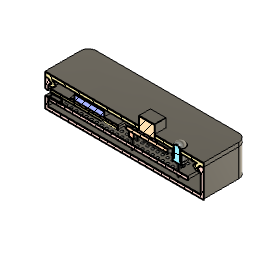
co2-sensor-d1-mini (Autodesk Fusion 360 design; units mm, degrees)
Autodesk Fusion 360 part; units mm, degrees
(part 1 of 2)
sketch "board" plane through (0, 0, 0) normal (0, 0, 1) x (1, 0, 0) in component "Board"
  line L0 (35, 15) -> (-35, 15)
  line L1 (-35, 15) -> (-35, -15)
  line L2 (-35, -15) -> (35, -15)
  line L3 (35, -15) -> (35, 15)
  line L4 (35, 15) -> (-35, -15) construction
  line L5 (-35, 15) -> (35, -15) construction
  dimension "d4" = 70
  dimension "d5" = 30
  constraint horizontal L0
  constraint perpendicular L0 L1
  constraint parallel L0 L2
  constraint parallel L1 L3
  constraint coincident L4 origin
  constraint coincident L5 origin
  measures "d4" distance of L1.end L2.end
  measures "d5" distance of L0.end L1.end
extrude "Extrude1" add sketch "board" along normal blind 1.5 makes body 1 in component "Board"
sketch "holes" plane through (0, 0, 1.5) normal (0, 0, 1) x (-1, 0, 0) in component "Board"
  line L0 (-35, 15) -> (-35, -15)
  line L1 (-35, -15) -> (35, -15)
  line L2 (35, -15) -> (35, 15)
  line L3 (35, 15) -> (-35, 15)
  line L4 (-29.5, -11.5) -> (29.5, -11.5) construction
  line L5 (29.5, -11.5) -> (29.5, 11.5) construction
  line L6 (29.5, 11.5) -> (-29.5, 11.5) construction
  line L7 (-29.5, 11.5) -> (-29.5, -11.5) construction
  line L8 (-29.5, -11.5) -> (29.5, 11.5) construction
  line L9 (29.5, -11.5) -> (-29.5, 11.5) construction
  line L10 (-33, -13.1) -> (33, -13.1) construction
  line L11 (33, -13.1) -> (33, 13.1) construction
  line L12 (33, 13.1) -> (-33, 13.1) construction
  line L13 (-33, 13.1) -> (-33, -13.1) construction
  line L14 (-33, -13.1) -> (33, 13.1) construction
  line L15 (33, -13.1) -> (-33, 13.1) construction
  circle A0 centre (33, -13.1) radius 1.2
  circle A1 centre (29.5, -11.5) radius 0.7
  dimension "d13" = 59
  dimension "d14" = 23
  dimension "d15" = 66
  dimension "d16" = 26.2
  dimension "d17" = 2.4
  dimension "d18" = 1.4
  constraint horizontal L4
  constraint perpendicular L4 L5
  constraint parallel L4 L6
  constraint parallel L5 L7
  constraint coincident L8 origin
  constraint coincident L9 origin
  constraint horizontal L10
  constraint perpendicular L10 L11
  constraint parallel L10 L12
  constraint parallel L11 L13
  constraint coincident L14 origin
  constraint coincident L15 origin
  constraint coincident L10.end L11.start
  constraint coincident L4.end L5.start
  measures "d13" distance of L5.end L6.end
  measures "d14" distance of L4.end L5.end
  measures "d15" distance of L11.end L12.end
  measures "d16" distance of L10.end L11.end
  measures "d17" diameter of A0
  measures "d18" diameter of A1
extrude "Extrude2" cut sketch "holes" against normal through all contours A0 bodies 1 in component "Board"
pattern_linear "R-Pattern1" count 2 spacing 66 along (1, 0, 0) count 2 spacing 26.2 along (0, -1, 0) of "Extrude2" in component "Board"
extrude "Extrude3" cut sketch "holes" against normal through all contours A1 bodies 1 in component "Board"
pattern_linear "R-Pattern2" count 24 spacing 2.5652 along (1, 0, 0) count 10 spacing 2.5556 along (0, -1, 0) of "Extrude3" in component "Board"
sketch "base" plane through (0, 0, 0) normal (0, 0, 1) x (1, 0, 0) in component "D1 Mini"
  line L0 (17.075, 12.8) -> (-17.075, 12.8)
  line L1 (-17.075, 12.8) -> (-17.075, -12.8)
  line L2 (-17.075, -12.8) -> (17.075, -12.8)
  line L3 (17.075, -12.8) -> (17.075, 12.8)
  line L4 (17.075, 12.8) -> (-17.075, -12.8) construction
  line L5 (-17.075, 12.8) -> (17.075, -12.8) construction
  dimension "d29" = 34.15
  dimension "d30" = 25.6
  constraint horizontal L0
  constraint perpendicular L0 L1
  constraint parallel L0 L2
  constraint parallel L1 L3
  constraint coincident L4 origin
  constraint coincident L5 origin
  measures "d29" distance of L1.end L2.end
  measures "d30" distance of L0.end L1.end
extrude "Extrude1'" add sketch "base" along normal blind 1.14 separate body makes body 2 in component "D1 Mini"
copy_body "Body->Comp1" bodies 2 removing the originals makes body 3 in component "base"
sketch "holes (2)" plane through (0, 0, 1.14) normal (0, 0, 1) x (-1, 0, 0) in component "D1 Mini"
  line L0 (-17.075, 12.8) -> (-17.075, -12.8)
  line L1 (-17.075, -12.8) -> (17.075, -12.8)
  line L2 (17.075, -12.8) -> (17.075, 12.8)
  line L3 (17.075, 12.8) -> (-17.075, 12.8)
  line L4 (-15, -11.5) -> (15, -11.5) construction
  line L5 (15, -11.5) -> (15, 11.5) construction
  line L6 (15, 11.5) -> (-15, 11.5) construction
  line L7 (-15, 11.5) -> (-15, -11.5) construction
  line L8 (-15, -11.5) -> (15, 11.5) construction
  line L9 (15, -11.5) -> (-15, 11.5) construction
  line L10 (8.375, -12.8) -> (8.375, 12.8) construction
  circle A0 centre (8.375, -11.5) radius 0.65
  dimension "d33" = 30
  dimension "d34" = 23
  dimension "d35" = 8.7
  dimension "d36" = 1.3
  constraint horizontal L4
  constraint perpendicular L4 L5
  constraint parallel L4 L6
  constraint parallel L5 L7
  constraint coincident L8 origin
  constraint coincident L9 origin
  constraint coincident L1 L10.start
  constraint coincident L3 L10.end
  constraint perpendicular L3 L10
  constraint coincident L4 A0.centre
  constraint coincident L10 A0.centre
  measures "d33" distance of L5.end L6.end
  measures "d34" distance of L4.end L5.end
  measures "d35" distance of L2 L10
  measures "d36" diameter of A0
extrude "Extrude1''" cut sketch "holes (2)" against normal through all contours A0 bodies 3 in component "base"
pattern_linear "R-Pattern1'" count 8 spacing 2.565 along (1, 0, 0) count 2 spacing 23 along (0, -1, 0) of "Extrude1''" in component "base"
sketch "Sketch1" plane through (0, 0, 1.14) normal (0, 0, 1) x (-1, 0, 0) in component "base (1)"
  circle A0 centre (-9.58, 11.5) radius 0.65
  circle A1 centre (-7.015, 11.5) radius 0.65
  circle A2 centre (-4.45, 11.5) radius 0.65
  circle A3 centre (-1.885, 11.5) radius 0.65
  circle A4 centre (0.68, 11.5) radius 0.65
  circle A5 centre (3.245, 11.5) radius 0.65
  circle A6 centre (5.81, 11.5) radius 0.65
  circle A7 centre (8.375, 11.5) radius 0.65
  circle A8 centre (-9.58, -11.5) radius 0.65
  circle A9 centre (-7.015, -11.5) radius 0.65
  circle A10 centre (-4.45, -11.5) radius 0.65
  circle A11 centre (-1.885, -11.5) radius 0.65
  circle A12 centre (0.68, -11.5) radius 0.65
  circle A13 centre (3.245, -11.5) radius 0.65
  circle A14 centre (5.81, -11.5) radius 0.65
  circle A15 centre (8.375, -11.5) radius 0.65
  line L0 (-17.075, 12.8) -> (-17.075, -12.8)
  line L1 (-17.075, -12.8) -> (17.075, -12.8)
  line L2 (17.075, -12.8) -> (17.075, 12.8)
  line L3 (17.075, 12.8) -> (-17.075, 12.8)
  line L4 (17.075, -8) -> (-6.925, -8)
  line L5 (-6.925, -8) -> (-6.925, 8)
  line L6 (-6.925, 8) -> (17.075, 8)
  line L7 (17.075, 8) -> (17.075, -8)
  line L8 (17.075, 0) -> (-6.925, 0) construction
  dimension "d44" = 24
  dimension "d45" = 16
  constraint horizontal L4
  constraint vertical L5
  constraint horizontal L6
  constraint vertical L7
  constraint coincident L2 L4.start
  constraint midpoint L2 L8.start
  constraint midpoint L5 L8.end
  constraint horizontal L8
  measures "d44" distance of L4.start L4.end
  measures "d45" distance of L4.start L6.end
extrude "Extrude1'''" add sketch "Sketch1" along normal blind 1 separate body contours L2 L4 L5 L6 L7 makes body 4 in component "base (1)"
sketch "Sketch1 (2)" plane through (0, 0, 2.14) normal (0, 0, 1) x (-1, 0, 0) in component "CPU (1)"
  line L0 (17.075, 8) -> (-6.925, 8)
  line L1 (-6.925, 8) -> (-6.925, -8)
  line L2 (-6.925, -8) -> (17.075, -8)
  line L3 (17.075, -8) -> (17.075, 8)
  line L4 (10.075, -8) -> (10.075, 8) construction
  line L5 (10.075, -6) -> (-4.925, -6)
  line L6 (-4.925, -6) -> (-4.925, 6)
  line L7 (-4.925, 6) -> (10.075, 6)
  line L8 (10.075, 6) -> (10.075, -6)
  line L9 (17.075, 0) -> (10.075, 0) construction
  line L10 (10.5763, -6.8) -> (11.3763, -6.8)
  line L11 (11.3763, -6.8) -> (11.3763, -4.8)
  line L12 (11.3763, -4.8) -> (10.5763, -4.8)
  line L13 (10.5763, -4.8) -> (10.5763, -6.8)
  line L14 (13.1321, -4.8) -> (10.3131, -4.8) construction
  line L15 (10.075, -8) -> (10.075, 8) construction
  dimension "d48" = 7
  dimension "d49" = 15
  dimension "d50" = 12
  dimension "d51" = 0.8
  dimension "d52" = 2
  dimension "d53" = 3.2
  constraint coincident L2 L4.start
  constraint coincident L0 L4.end
  constraint perpendicular L0 L4
  constraint horizontal L5
  constraint vertical L6
  constraint horizontal L7
  constraint vertical L8
  constraint coincident L4 L5.start
  constraint midpoint L3 L9.start
  constraint midpoint L8 L9.end
  constraint horizontal L9
  constraint horizontal L10
  constraint vertical L11
  constraint horizontal L12
  constraint vertical L13
  constraint horizontal L14
  constraint collinear L12 L14
  constraint perpendicular L0 L15
  measures "d48" distance of L3 L4
  measures "d49" distance of L5.start L5.end
  measures "d50" distance of L5.start L7.end
  measures "d51" distance of L10.start L10.end
  measures "d52" distance of L10.start L12.end
  measures "d53" distance of L2 L14
extrude "Extrude1''''" add sketch "Sketch1 (2)" along normal blind 2.75 separate body contours L5 L6 L7 L8 makes body 5 in component "CPU (1)"
extrude "Extrude2'" add sketch "Sketch1 (2)" along normal blind 0.2 separate body contours L10 L11 L12 L13 makes body 6 in component "CPU (1)"
sketch "Sketch1 (3)" plane through (0, 0, 0) normal (0, 0, 1) x (1, 0, 0) in component "pin"
  line L0 (1.2563, 1.2563) -> (-1.2563, 1.2563)
  line L1 (-1.2563, 1.2563) -> (-1.2563, -1.2563)
  line L2 (-1.2563, -1.2563) -> (1.2563, -1.2563)
  line L3 (1.2563, -1.2563) -> (1.2563, 1.2563)
  line L4 (1.2563, 1.2563) -> (-1.2563, -1.2563) construction
  line L5 (-1.2563, 1.2563) -> (1.2563, -1.2563) construction
  line L6 (-0.34, 0.34) -> (0.34, 0.34)
  line L7 (0.34, 0.34) -> (0.34, -0.34)
  line L8 (0.34, -0.34) -> (-0.34, -0.34)
  line L9 (-0.34, -0.34) -> (-0.34, 0.34)
  line L10 (-0.34, 0.34) -> (0.34, -0.34) construction
  line L11 (0.34, 0.34) -> (-0.34, -0.34) construction
  dimension "d59" = 2.5125
  dimension "d60" = 2.5125
  dimension "d61" = 0.68
  dimension "d62" = 0.68
  constraint horizontal L0
  constraint perpendicular L0 L1
  constraint parallel L0 L2
  constraint parallel L1 L3
  constraint coincident L4 origin
  constraint coincident L5 origin
  constraint horizontal L6
  constraint perpendicular L6 L7
  constraint parallel L6 L8
  constraint parallel L7 L9
  constraint coincident L10 origin
  constraint coincident L11 origin
  measures "d59" distance of L1.end L2.end
  measures "d60" distance of L0.end L1.end
  measures "d61" distance of L7.end L8.end
  measures "d62" distance of L6.end L7.end
extrude "Extrude1'''''" add sketch "Sketch1 (3)" along normal blind 11.1 separate body contours L6 L7 L8 L9 makes body 7 in component "pin"
copy_body "CutPasteBodies1" bodies 7 removing the originals makes body 8 in component "pin (1)"
extrude "Extrude1''''''" add sketch "Sketch1 (3)" along normal blind 2.65 separate body makes body 9 in component "shroud"
chamfer "Chamfer1" distance 0.2 angle 45 4 edges at (-1.2563, -1.2563, 1.325) (1.2563, -1.2563, 1.325) (1.2563, 1.2563, 1.325) (-1.2563, 1.2563, 1.325) on bodies 9 in component "shroud"
sketch "Sketch2" plane through (0, 0, 0) normal (0, 1, 0) x (1, 0, 0) in component "pin"
  line L0 (-3, 5.8) -> (3.7, 5.8) construction
  dimension "d68" = 5.8
  constraint horizontal L0
  measures "d68" distance of L0 origin
sketch "Sketch1 (4)" plane through (0, 0, 0) normal (0, 0, 1) x (1, 0, 0) in component "pin (2)"
  line L0 (1.2563, 1.2563) -> (-1.2563, 1.2563)
  line L1 (-1.2563, 1.2563) -> (-1.2563, -1.2563)
  line L2 (-1.2563, -1.2563) -> (1.2563, -1.2563)
  line L3 (1.2563, -1.2563) -> (1.2563, 1.2563)
  line L4 (1.2563, 1.2563) -> (-1.2563, -1.2563) construction
  line L5 (-1.2563, 1.2563) -> (1.2563, -1.2563) construction
  line L6 (-0.34, 0.34) -> (0.34, 0.34)
  line L7 (0.34, 0.34) -> (0.34, -0.34)
  line L8 (0.34, -0.34) -> (-0.34, -0.34)
  line L9 (-0.34, -0.34) -> (-0.34, 0.34)
  line L10 (-0.34, 0.34) -> (0.34, -0.34) construction
  line L11 (0.34, 0.34) -> (-0.34, -0.34) construction
  dimension "d59_1" = 2.5125
  dimension "d60_1" = 2.5125
  dimension "d61_1" = 0.68
  dimension "d62_1" = 0.68
  constraint horizontal L0
  constraint perpendicular L0 L1
  constraint parallel L0 L2
  constraint parallel L1 L3
  constraint coincident L4 origin
  constraint coincident L5 origin
  constraint horizontal L6
  constraint perpendicular L6 L7
  constraint parallel L6 L8
  constraint parallel L7 L9
  constraint coincident L10 origin
  constraint coincident L11 origin
  measures "d59_1" distance of L1.end L2.end
  measures "d60_1" distance of L0.end L1.end
  measures "d61_1" distance of L7.end L8.end
  measures "d62_1" distance of L6.end L7.end
extrude "Extrude1'''''''" add sketch "Sketch1 (4)" along normal blind 11.1 separate body contours L6 L7 L8 L9 makes body 10 in component "pin (2)"
copy_body "CutPasteBodies1'" bodies 10 removing the originals makes body 11 in component "pin (1) (1)"
extrude "Extrude1''''''''" add sketch "Sketch1 (4)" along normal blind 2.65 separate body makes body 12 in component "shroud (1)"
chamfer "Chamfer1'" distance 0.2 angle 45 4 edges at (-1.2563, -1.2563, 1.325) (1.2563, -1.2563, 1.325) (1.2563, 1.2563, 1.325) (-1.2563, 1.2563, 1.325) on bodies 12 in component "shroud (1)"
sketch "Sketch2 (2)" plane through (0, 0, 0) normal (0, 1, 0) x (1, 0, 0) in component "pin (2)"
  line L0 (-3, 5.8) -> (3.7, 5.8) construction
  dimension "d68_1" = 5.8
  constraint horizontal L0
  measures "d68_1" distance of L0 origin
pattern_linear "00000000-0000-0000-0000-000000000000" [suppressed] in component "pins"
sketch "Sketch1 (5)" plane through (17.075, 0, 0) normal (1, 0, 0) x (0, 1, 0) in component "USB port"
  line L0 (-12.8, 0) -> (12.8, 0)
  line L1 (12.8, 0) -> (12.8, 1.14)
  line L2 (12.8, 1.14) -> (-12.8, 1.14)
  line L3 (-12.8, 1.14) -> (-12.8, 0)
  line L4 (-3.75, 0) -> (3.75, 0)
  line L5 (3.75, 0) -> (3.75, -3)
  line L6 (3.75, -3) -> (-3.75, -3)
  line L7 (-3.75, -3) -> (-3.75, 0)
  line L8 (0, 0) -> (0, -3) construction
  dimension "d73" = 7.5
  dimension "d74" = 3
  constraint horizontal L4
  constraint vertical L5
  constraint horizontal L6
  constraint vertical L7
  constraint coincident L0 L4.start
  constraint coincident L8.start origin
  constraint midpoint L6 L8.end
  constraint vertical L8
  measures "d73" distance of L4.start L4.end
  measures "d74" distance of L4.start L6.end
extrude "Extrude1'''''''''" add sketch "Sketch1 (5)" against normal blind 5.9 separate body contours L0 L4 L5 L6 L7 makes body 13 in component "USB port"
shell "Shell1" thickness 0.45 removed faces 1 at (17.075, -1.25, -1) on bodies 13 in component "USB port"
sketch "base (2)" plane through (0, 0, 0) normal (0, 0, 1) x (1, 0, 0) in component "board"
  line L0 (-10, 10) -> (10, 10)
  line L1 (10, 10) -> (10, -10)
  line L2 (10, -10) -> (-10, -10)
  line L3 (-10, -10) -> (-10, 10)
  line L4 (-10, 10) -> (10, -10) construction
  line L5 (10, 10) -> (-10, -10) construction
  dimension "d78" = 20
  dimension "d79" = 20
  constraint horizontal L0
  constraint perpendicular L0 L1
  constraint parallel L0 L2
  constraint parallel L1 L3
  constraint coincident L4 origin
  constraint coincident L5 origin
  measures "d78" distance of L1.end L2.end
  measures "d79" distance of L0.end L1.end
extrude "Extrude1''''''''''" add sketch "base (2)" along normal blind 1.7 separate body makes body 14 in component "board"
sketch "Sketch1 (6)" plane through (0, 0, 1.7) normal (0, 0, 1) x (-1, 0, 0) in component "base (2)"
  line L0 (10, 10) -> (-10, 10)
  line L1 (-10, 10) -> (-10, -10)
  line L2 (-10, -10) -> (10, -10)
  line L3 (10, -10) -> (10, 10)
  line L4 (5.085, -5.085) -> (-5.085, -5.085)
  line L5 (-5.085, -5.085) -> (-5.085, 5.085)
  line L6 (-5.085, 5.085) -> (5.085, 5.085)
  line L7 (5.085, 5.085) -> (5.085, -5.085)
  line L8 (5.085, -5.085) -> (-5.085, 5.085) construction
  line L9 (-5.085, -5.085) -> (5.085, 5.085) construction
  dimension "d82" = 10.17
  dimension "d83" = 10.17
  constraint horizontal L4
  constraint perpendicular L4 L5
  constraint parallel L4 L6
  constraint parallel L5 L7
  constraint coincident L8 origin
  constraint coincident L9 origin
  measures "d82" distance of L5.end L6.end
  measures "d83" distance of L4.end L5.end
extrude "Extrude1'''''''''''" add sketch "Sketch1 (6)" along normal blind 1 separate body contours L4 L5 L6 L7 makes body 15 in component "base (2)"
sketch "Sketch1 (7)" plane through (0, 0, 2.7) normal (0, 0, 1) x (-1, 0, 0) in component "housing"
  line L0 (5.085, 5.085) -> (-5.085, 5.085)
  line L1 (-5.085, 5.085) -> (-5.085, -5.085)
  line L2 (-5.085, -5.085) -> (5.085, -5.085)
  line L3 (5.085, -5.085) -> (5.085, 5.085)
  line L4 (4, -4) -> (-4, -4)
  line L5 (-4, -4) -> (-4, 4)
  line L6 (-4, 4) -> (4, 4)
  line L7 (4, 4) -> (4, -4)
  line L8 (4, -4) -> (-4, 4) construction
  line L9 (-4, -4) -> (4, 4) construction
  dimension "d86" = 8
  dimension "d87" = 8
  constraint horizontal L4
  constraint perpendicular L4 L5
  constraint parallel L4 L6
  constraint parallel L5 L7
  constraint coincident L8 origin
  constraint coincident L9 origin
  measures "d86" distance of L5.end L6.end
  measures "d87" distance of L4.end L5.end
extrude "Extrude1''''''''''''" add sketch "Sketch1 (7)" along normal blind 6.3 separate body contours L4 L5 L6 L7 makes body 16 in component "housing"
fillet "Fillet1" radius 0.2 8 edges at (-4, -4, 5.85) (4, -4, 5.85) (0, -4, 9) (4, 0, 9) (-4, 0, 9) (4, 4, 5.85) (0, 4, 9) (-4, 4, 5.85) on bodies 16 in component "housing"
sketch "holes (3)" plane through (0, 0, 1.7) normal (0, 0, 1) x (-1, 0, 0) in component "board"
  line L0 (10, 10) -> (-10, 10)
  line L1 (-10, 10) -> (-10, -10)
  line L2 (-10, -10) -> (10, -10)
  line L3 (10, -10) -> (10, 10)
  arc A0 (2.1, -10) -> (-2.1, -10) centre (0, -10) ccw
  arc A1 (10, -2.1) -> (10, 2.1) centre (10, 0) ccw
  circle A2 centre (10, 0) radius 0.9
  line L4 (7.88, -10) -> (7.88, 10) construction
  line L5 (10, -3.8475) -> (-10, -3.8475) construction
  circle A3 centre (7.88, -3.8475) radius 0.65
  line L6 (10, 7.5) -> (-10, 7.5) construction
  line L7 (5.75, -10) -> (5.75, 10) construction
  line L8 (5.75, 7.5) -> (8.25, 7.5)
  line L9 (8.25, 7.5) -> (8.25, 8.5)
  line L10 (8.25, 8.5) -> (5.75, 8.5)
  line L11 (5.75, 8.5) -> (5.75, 7.5)
  line L12 (10, 3.8475) -> (-10, 3.8475) construction
  line L13 (-4.0475, -10) -> (-4.0475, -3.8475) construction
  line L14 (-4.2731, 3.8475) -> (-4.2731, 10) construction
  dimension "d92" = 2.1
  dimension "d93" = 2.1
  dimension "d94" = 1.8
  dimension "d95" = 2.12
  dimension "d97" = 1.3
  dimension "d98" = 2.5
  dimension "d99" = 4.25
  dimension "d100" = 2.5
  dimension "d101" = 1
  dimension "d115" = 7.695
  constraint coincident L2 A0.start
  constraint midpoint L2 A0.centre
  constraint coincident L3 A1.start
  constraint midpoint L3 A1.centre
  constraint concentric A1 A2
  constraint coincident L2 L4.start
  constraint coincident L0 L4.end
  constraint perpendicular L0 L4
  constraint coincident L3 L5.start
  constraint coincident L1 L5.end
  constraint perpendicular L1 L5
  constraint coincident L4 A3.centre
  constraint coincident L5 A3.centre
  constraint coincident L3 L6.start
  constraint coincident L1 L6.end
  constraint perpendicular L1 L6
  constraint coincident L2 L7.start
  constraint coincident L0 L7.end
  constraint perpendicular L0 L7
  constraint horizontal L8
  constraint vertical L9
  constraint horizontal L10
  constraint vertical L11
  constraint coincident L6 L8.start
  constraint coincident L7 L8.start
  constraint coincident L3 L12.start
  constraint coincident L1 L12.end
  constraint perpendicular L1 L12
  constraint coincident L2 L13.start
  constraint coincident L5 L13.end
  constraint perpendicular L5 L13
  constraint coincident L12 L14.start
  constraint perpendicular L0 L14
  constraint equal L13 L14
  constraint coincident L0 L14.end
  measures "d92" radius of A0
  measures "d93" radius of A1
  measures "d94" diameter of A2
  measures "d95" distance of L3 L4
  measures "d97" diameter of A3
  measures "d98" distance of L0 L6
  measures "d99" distance of L3 L7
  measures "d100" distance of L8.start L8.end
  measures "d101" distance of L8.start L10.end
  measures "d115" distance of L5 L12
extrude "Extrude2''" cut sketch "holes (3)" against normal through all contours L2 A0 bodies 14 in component "board"
ref_plane "WorkPlane1" through (6.05, 0, 0.85) normal (0, 1, 0) x (-1, 0, 0) in component "board"
mirror "Mirror1" about plane through (6.05, 0, 0.85) normal (0, 1, 0) of "Extrude2''" in component "board"
extrude "Extrude3'" add sketch "holes (3)" against normal up to surface (1.7 mm away) contours L3 A1 A2 bodies 14 in component "board"
extrude "Extrude4" cut sketch "holes (3)" against normal through all contours L3 A2 picked at (9.4663, -0.2095) bodies 14 in component "board"
ref_plane "WorkPlane2" through (0, 6.05, 0.85) normal (-1, 0, 0) x (0, -1, 0) in component "board"
mirror "Mirror2" about plane through (0, 6.05, 0.85) normal (-1, 0, 0) of "Extrude3'", "Extrude4" in component "board"
extrude "Extrude5" cut sketch "holes (3)" against normal through all contours A3 bodies 14 in component "board"
pattern_linear "R-Pattern1''" count 4 spacing 2.565 along (0, -1, 0) of "Extrude5" in component "board"
extrude "Extrude6" add sketch "holes (3)" along normal blind 0.8 separate body contours L8 L9 L10 L11 makes body 17 in component "board"
sketch "Sketch1 (8)" plane through (0, 10, 0) normal (0, 1, 0) x (-1, 0, 0) in component "connectort"
  line L0 (-2.1, 0) -> (-2.1, 1.7)
  line L1 (-2.1, 1.7) -> (-10, 1.7)
  line L2 (-10, 1.7) -> (-10, 0)
  line L3 (-10, 0) -> (-2.1, 0)
  line L4 (6, 0) -> (-6, 0)
  line L5 (-6, 0) -> (-6, -5.4)
  line L6 (-6, -5.4) -> (6, -5.4)
  line L7 (6, -5.4) -> (6, 0)
  line L8 (0, 0) -> (0, -5.4) construction
  dimension "d118" = 12
  dimension "d119" = 5.4
  constraint horizontal L4
  constraint vertical L5
  constraint horizontal L6
  constraint vertical L7
  constraint coincident L8.start origin
  constraint midpoint L6 L8.end
  constraint vertical L8
  constraint coincident L8.start L4
  measures "d118" distance of L4.start L4.end
  measures "d119" distance of L4.start L6.end
extrude "Extrude1'''''''''''''" add sketch "Sketch1 (8)" against normal blind 7.7 separate body contours L3 L4 L5 L6 L7 makes body 18 in component "connectort"
shell "Shell1'" thickness 0.6 removed faces 1 at (0.7, 10, -3.6) on bodies 18 in component "connectort"
sketch "Sketch1 (9)" plane through (0, 0, 0) normal (0, 0, 1) x (1, 0, 0) in component "pin (3)"
  line L0 (1.2563, 1.2563) -> (-1.2563, 1.2563)
  line L1 (-1.2563, 1.2563) -> (-1.2563, -1.2563)
  line L2 (-1.2563, -1.2563) -> (1.2563, -1.2563)
  line L3 (1.2563, -1.2563) -> (1.2563, 1.2563)
  line L4 (1.2563, 1.2563) -> (-1.2563, -1.2563) construction
  line L5 (-1.2563, 1.2563) -> (1.2563, -1.2563) construction
  line L6 (-0.34, 0.34) -> (0.34, 0.34)
  line L7 (0.34, 0.34) -> (0.34, -0.34)
  line L8 (0.34, -0.34) -> (-0.34, -0.34)
  line L9 (-0.34, -0.34) -> (-0.34, 0.34)
  line L10 (-0.34, 0.34) -> (0.34, -0.34) construction
  line L11 (0.34, 0.34) -> (-0.34, -0.34) construction
  dimension "d59_2" = 2.5125
  dimension "d60_2" = 2.5125
  dimension "d61_2" = 0.68
  dimension "d62_2" = 0.68
  constraint horizontal L0
  constraint perpendicular L0 L1
  constraint parallel L0 L2
  constraint parallel L1 L3
  constraint coincident L4 origin
  constraint coincident L5 origin
  constraint horizontal L6
  constraint perpendicular L6 L7
  constraint parallel L6 L8
  constraint parallel L7 L9
  constraint coincident L10 origin
  constraint coincident L11 origin
  measures "d59_2" distance of L1.end L2.end
  measures "d60_2" distance of L0.end L1.end
  measures "d61_2" distance of L7.end L8.end
  measures "d62_2" distance of L6.end L7.end
extrude "Extrude1''''''''''''''" add sketch "Sketch1 (9)" along normal blind 11.1 separate body contours L6 L7 L8 L9 makes body 19 in component "pin (3)"
copy_body "CutPasteBodies1''" bodies 19 removing the originals makes body 20 in component "pin (1) (2)"
extrude "Extrude1'''''''''''''''" add sketch "Sketch1 (9)" along normal blind 2.65 separate body makes body 21 in component "shroud (2)"
chamfer "Chamfer1''" distance 0.2 angle 45 4 edges at (-1.2563, -1.2563, 1.325) (1.2563, -1.2563, 1.325) (1.2563, 1.2563, 1.325) (-1.2563, 1.2563, 1.325) on bodies 21 in component "shroud (2)"
sketch "Sketch2 (3)" plane through (0, 0, 0) normal (0, 1, 0) x (1, 0, 0) in component "pin (3)"
  line L0 (-3, 5.8) -> (3.7, 5.8) construction
  dimension "d68_2" = 5.8
  constraint horizontal L0
  measures "d68_2" distance of L0 origin
pattern_linear "00000000-0000-0000-0000-000000000000'" [suppressed] in component "pins (1)"
sketch "Sketch2 (4)" plane through (0, 0, 0) normal (0, 1, 0) x (1, 0, 0) in component "RGBLED"
  line L0 (0, 0) -> (-2.9, 0)
  line L1 (-2.9, 0) -> (-2.9, -0.05)
  line L2 (-2.9, 0) -> (-2.9, -1)
  line L3 (-2.9, -1) -> (-2.5, -1)
  line L4 (-4, -8.35) -> (5.4561, -8.35) construction
  line L5 (0, 0) -> (0, -8.35)
  line L6 (-3.9559, -6.7) -> (5.5441, -6.7) construction
  line L7 (-2.5, -1) -> (-2.5, -6.7)
  arc A0 (-2.5, -6.7) -> (0, -8.35) centre (0, -5.6311) ccw
  dimension "d127" = 2.9
  dimension "d128" = 1
  dimension "d129" = 0.4
  dimension "d131" = 8.35
  dimension "d232" = 6.7
  constraint coincident L0.start L5.start
  constraint horizontal L0
  constraint perpendicular L0 L1
  constraint perpendicular L0 L2
  constraint perpendicular L2 L3
  constraint horizontal L4
  constraint coincident L4 L5.end
  constraint perpendicular L4 L5
  constraint horizontal L6
  constraint coincident L6 L7.end
  constraint perpendicular L6 L7
  constraint tangent L4 A0
  measures "d127" distance of L0.start L0.end
  measures "d128" distance of L0.end L2.end
  measures "d129" distance of L2.end L3.end
  measures "d131" distance of L0 L4
  measures "d232" distance of L0 L6
revolve "Revolve1" add sketch "Sketch2 (4)" angle 360 about axis through (0, 0, 0) along (0, 0, 1) separate body makes body 22 in component "RGBLED"
sketch "Sketch3" plane through (0, 0, 0) normal (0, 0, -1) x (1, 0, 0) in component "RGBLED"
  circle A0 centre (0, 0) radius 2.9
  line L0 (0, 2.2) -> (0, -2.2) construction
  line L1 (0, 2.2) -> (0, 2.9) construction
  line L2 (0, -2.2) -> (0, -2.9) construction
  line L3 (0.33, 2.53) -> (-0.33, 2.53)
  line L4 (-0.33, 2.53) -> (-0.33, 1.87)
  line L5 (-0.33, 1.87) -> (0.33, 1.87)
  line L6 (0.33, 1.87) -> (0.33, 2.53)
  line L7 (0.33, 2.53) -> (-0.33, 1.87) construction
  line L8 (-0.33, 2.53) -> (0.33, 1.87) construction
  point P0 (0, 2.2)
  dimension "d133" = 4.4
  dimension "d134" = 0.66
  dimension "d135" = 0.66
  constraint vertical L0
  constraint coincident A0 L1.end
  constraint parallel L0 L1
  constraint coincident A0 L2.end
  constraint parallel L0 L2
  constraint equal L1 L2
  constraint horizontal L3
  constraint perpendicular L3 L4
  constraint parallel L3 L5
  constraint parallel L4 L6
  constraint coincident L7 P0
  constraint coincident L8 P0
  constraint coincident P0 L0.start
  measures "d133" distance of P0 L0.end
  measures "d134" distance of L4.end L5.end
  measures "d135" distance of L3.end L4.end
extrude "Extrude1''''''''''''''''" add sketch "Sketch3" along normal blind 7 separate body contours L3 L4 L5 L6 makes body 23 in component "RGBLED"
pattern_linear "R-Pattern1'''" count 4 spacing 1.4 along (0, 1, 0) of bodies 23 makes body 24 at (-0.11, -0.47, -2.3333) makes body 25 at (-0.11, 0.93, -2.3333) makes body 26 at (-0.11, 2.33, -2.3333) in component "RGBLED"
sketch "case" plane through (0, 0, 0) normal (0, 0, 1) x (1, 0, 0) in component "base (3)"
  line L0 (40, 20) -> (-40, 20)
  line L1 (-40, 20) -> (-40, -20)
  line L2 (-40, -20) -> (40, -20)
  line L3 (40, -20) -> (40, 20)
  line L4 (40, 20) -> (-40, -20) construction
  line L5 (-40, 20) -> (40, -20) construction
  dimension "d169" = 80
  dimension "d170" = 40
  constraint horizontal L0
  constraint perpendicular L0 L1
  constraint parallel L0 L2
  constraint parallel L1 L3
  constraint coincident L4 origin
  constraint coincident L5 origin
  measures "d169" distance of L1.end L2.end
  measures "d170" distance of L0.end L1.end
extrude "Extrude1'''''''''''''''''" add sketch "case" along normal blind 14 separate body makes body 27 in component "base (3)"
fillet "Fillet1'" radius 4 4 edges at (-40, -20, 7) (-40, 20, 7) (40, -20, 7) (40, 20, 7) on bodies 27 in component "base (3)"
shell "Shell1''" thickness 1.5 removed faces 1 at (12, -6.6667, 14) on bodies 27 in component "base (3)"
sketch "nubs" plane through (-38.5, 0, 0) normal (1, 0, 0) x (0, 1, 0) in component "base (3)"
  line L0 (16, 1.5) -> (16, 14)
  line L1 (16, 14) -> (-16, 14)
  line L2 (-16, 14) -> (-16, 1.5)
  line L3 (-16, 1.5) -> (16, 1.5)
  line L4 (-10, 14) -> (10, 14)
  line L5 (10, 14) -> (10, 11)
  line L6 (10, 11) -> (-10, 11)
  line L7 (-10, 11) -> (-10, 14)
  line L8 (0, 14) -> (0, 11) construction
  dimension "d176" = 20
  dimension "d177" = 3
  constraint horizontal L4
  constraint vertical L5
  constraint horizontal L6
  constraint vertical L7
  constraint coincident L1 L4.start
  constraint midpoint L1 L8.start
  constraint midpoint L6 L8.end
  constraint vertical L8
  measures "d176" distance of L4.start L4.end
  measures "d177" distance of L4.start L6.end
extrude "Extrude2'''" add sketch "nubs" along normal blind 3 draft -45 contours L1 L4 L5 L6 L7 bodies 27 in component "base (3)"
ref_plane "WorkPlane1" through (0, 0, 7) normal (1, 0, 0) x (0, 1, 0) in component "base (3)"
mirror "Mirror1'" about plane through (0, 0, 7) normal (1, 0, 0) of "Extrude2'''" in component "base (3)"
sketch "Sketch1 (10)" plane through (0, 0, 14) normal (0, 0, 1) x (-1, 0, 0) in component "lid"
  arc A0 (36, -18.5) -> (38.5, -16) centre (36, -16) ccw
  line L0 (36, -18.5) -> (-36, -18.5)
  arc A1 (-38.5, -16) -> (-36, -18.5) centre (-36, -16) ccw
  line L1 (-38.5, -16) -> (-38.5, -10)
  line L2 (-38.5, -10) -> (-38.5, 10)
  line L3 (-38.5, 10) -> (-38.5, 16)
  arc A2 (-36, 18.5) -> (-38.5, 16) centre (-36, 16) ccw
  line L4 (-36, 18.5) -> (36, 18.5)
  arc A3 (38.5, 16) -> (36, 18.5) centre (36, 16) ccw
  line L5 (38.5, 16) -> (38.5, 10)
  line L6 (38.5, 10) -> (38.5, -10)
  line L7 (38.5, -10) -> (38.5, -16)
  arc A4 (-40, -16) -> (-36, -20) centre (-36, -16) ccw
  line L8 (-36, -20) -> (36, -20)
  arc A5 (36, -20) -> (40, -16) centre (36, -16) ccw
  line L9 (40, -16) -> (40, 16)
  arc A6 (40, 16) -> (36, 20) centre (36, 16) ccw
  line L10 (36, 20) -> (-36, 20)
  arc A7 (-36, 20) -> (-40, 16) centre (-36, 16) ccw
  line L11 (-40, 16) -> (-40, -16)
extrude "Extrude1''''''''''''''''''" add sketch "Sketch1 (10)" along normal blind 2 separate body contours A0 L0 A1 L1 L2 L3 A2 L4 A3 L5 L6 L7 | A4 L8 A5 L9 A6 L10 A7 L11 makes body 28 in component "lid"
sketch "Sketch2 (5)" plane through (0, 0, 14) normal (0, 0, -1) x (1, 0, 0) in component "lid"
  line L0 (40, -16) -> (40, 16)
  arc A0 (40, 16) -> (36, 20) centre (36, 16) ccw
  line L1 (36, 20) -> (-36, 20)
  arc A1 (-36, 20) -> (-40, 16) centre (-36, 16) ccw
  line L2 (-40, 16) -> (-40, -16)
  arc A2 (-40, -16) -> (-36, -20) centre (-36, -16) ccw
  line L3 (-36, -20) -> (36, -20)
  arc A3 (36, -20) -> (40, -16) centre (36, -16) ccw
  arc A4 (-38.3, -16) -> (-36, -18.3) centre (-36, -16) ccw
  line L4 (-36, -18.3) -> (36, -18.3)
  arc A5 (36, -18.3) -> (38.3, -16) centre (36, -16) ccw
  line L5 (38.3, -16) -> (38.3, 16)
  arc A6 (38.3, 16) -> (36, 18.3) centre (36, 16) ccw
  line L6 (36, 18.3) -> (-36, 18.3)
  arc A7 (-36, 18.3) -> (-38.3, 16) centre (-36, 16) ccw
  line L7 (-38.3, 16) -> (-38.3, -16)
extrude "Extrude2''''" add sketch "Sketch2 (5)" along normal blind 3 contours A4 L4 A5 L5 A6 L6 A7 L7 bodies 28 in component "lid"
extrude "Extrude3''" cut sketch "nubs" along normal blind 3 draft -45 from surface at 0.2 contours L1 L4 L5 L6 L7 bodies 28 in component "lid"
chamfer "Chamfer1'''" distance 0.6 angle 45 1 edges at (-38.3, 0, 11) on bodies 28 in component "lid"
mirror "Mirror1''" about plane through (0, 0, 7) normal (1, 0, 0) of "Extrude3''" in component "lid"
shell "Shell1'''" thickness 1.5 removed faces 1 at (12.9667, 3.1333, 11) on bodies 28 in component "lid"
chamfer "Chamfer2" distance 0.6 angle 45 1 edges at (38.3, 0, 11) on bodies 28 in component "lid"
sketch "post bases" plane through (0, 0, 1.5) normal (0, 0, 1) x (-1, 0, 0) in component "base (3)"
  arc A0 (-38.5, -16) -> (-36, -18.5) centre (-36, -16) ccw
  line L0 (-36, -18.5) -> (36, -18.5)
  arc A1 (36, -18.5) -> (38.5, -16) centre (36, -16) ccw
  line L1 (38.5, -16) -> (38.5, 16)
  arc A2 (38.5, 16) -> (36, 18.5) centre (36, 16) ccw
  line L2 (36, 18.5) -> (-36, 18.5)
  arc A3 (-36, 18.5) -> (-38.5, 16) centre (-36, 16) ccw
  line L3 (-38.5, 16) -> (-38.5, -16)
  circle A4 centre (36, -13.1) radius 1.7
  line L4 (36, -13.1) -> (-30, -13.1) construction
  line L5 (-30, -13.1) -> (-30, 13.1) construction
  line L6 (-30, 13.1) -> (36, 13.1) construction
  line L7 (36, 13.1) -> (36, -13.1) construction
  line L8 (0, -18.5) -> (3, -13.1) construction
  line L9 (0, 18.5) -> (3, 13.1) construction
  line L10 (36, -18.5) -> (36, 18.5) construction
  dimension "d197" = 3.4
  dimension "d208" = 66
  dimension "d209" = 26.2
  dimension "d211" = 2.5
  constraint horizontal L4
  constraint vertical L5
  constraint horizontal L6
  constraint vertical L7
  constraint midpoint L0 L8.start
  constraint midpoint L4 L8.end
  constraint midpoint L2 L9.start
  constraint midpoint L6 L9.end
  constraint equal L8 L9
  constraint coincident L0 A1.start
  constraint coincident L2 A2.end
  constraint perpendicular L2 L10
  constraint collinear L7 L10
  constraint coincident A4.centre L4.start
  measures "d197" diameter of A4
  measures "d208" distance of A4.centre L4.end
  measures "d209" distance of A4.centre L6.end
  measures "d211" distance of L1 L10
extrude "Extrude3'''" add sketch "post bases" along normal blind 3 separate body contours A4 makes body 29 in component "base (3)"
sketch "posts (1)" plane through (0, 0, 4.5) normal (0, 0, 1) x (-1, 0, 0) in component "base (3)"
  circle A0 centre (36, -13.1) radius 1.7
  circle A1 centre (36, -13.1) radius 1.1
  dimension "d201" = 2.2
  constraint concentric A0 A1
  measures "d201" diameter of A1
extrude "Extrude4'" add sketch "posts (1)" along normal blind 1.5 contours A1 bodies 27 29 in component "base (3)"
pattern_linear "R-Pattern1''''" count 2 spacing 66 along (1, 0, 0) count 2 spacing 26.2 along (0, -1, 0) of bodies 29 makes body 30 at (28.3021, 13.1847, 3.5) makes body 31 at (-37.6979, -13.0153, 3.5) makes body 32 at (28.3021, -13.0153, 3.5) in component "base (3)"
sketch "Sketch1 (11)" plane through (-40, 0, 0) normal (-1, 0, 0) x (0, -1, 0) in component "Case"
  line L0 (-16, 14) -> (-16, 0)
  line L1 (-16, 0) -> (16, 0)
  line L2 (16, 0) -> (16, 14)
  line L3 (16, 14) -> (-16, 14)
  line L4 (-3.8265, 8.7265) -> (3.853, 8.7265)
  line L5 (3.853, 8.7265) -> (3.853, 5.6653)
  line L6 (3.853, 5.6653) -> (-3.8265, 5.6653)
  line L7 (-3.8265, 5.6653) -> (-3.8265, 8.7265)
  constraint horizontal L4
  constraint vertical L5
  constraint horizontal L6
  constraint vertical L7
extrude "Extrude5'" cut sketch "Sketch1 (11)" against normal up to surface (1.5 mm away) contours L4 L5 L6 L7 bodies 27 in component "base (3)"
fillet "Fillet2" radius 0.3 4 edges at (-40, 3.8265, 7.1959) (-40, -0.0133, 8.7265) (-40, -3.853, 7.1959) (-40, -0.0133, 5.6653) on bodies 27 in component "base (3)"
sketch "ports - top" plane through (0, 0, 16) normal (0, 0, 1) x (-1, 0, 0) in component "lid"
  line L0 (-40, 16) -> (-40, -16)
  arc A0 (-40, -16) -> (-36, -20) centre (-36, -16) ccw
  line L1 (-36, -20) -> (36, -20)
  arc A1 (36, -20) -> (40, -16) centre (36, -16) ccw
  line L2 (40, -16) -> (40, 16)
  arc A2 (40, 16) -> (36, 20) centre (36, 16) ccw
  line L3 (36, 20) -> (-36, 20)
  arc A3 (-36, 20) -> (-40, 16) centre (-36, 16) ccw
  arc A4 (-15.3, -3.85) -> (-15.1, -4.05) centre (-15.1, -3.85) ccw
  arc A5 (-7.5, -4.05) -> (-7.3, -3.85) centre (-7.5, -3.85) ccw
  arc A6 (-15.1, 3.95) -> (-15.3, 3.75) centre (-15.1, 3.75) ccw
  arc A7 (-7.3, 3.75) -> (-7.5, 3.95) centre (-7.5, 3.75) ccw
  line L4 (-15.3, -3.85) -> (-15.3, 3.75)
  line L5 (-15.1, 3.95) -> (-7.5, 3.95)
  line L6 (-7.3, 3.75) -> (-7.3, -3.85)
  line L7 (-7.5, -4.05) -> (-15.1, -4.05)
  circle A8 centre (-26.5, 11.5) radius 0.7
  circle A9 centre (-23.9348, 11.5) radius 0.7
  circle A10 centre (-21.3696, 11.5) radius 0.7
  circle A11 centre (-18.8043, 11.5) radius 0.7
  circle A12 centre (-16.2391, 11.5) radius 0.7
  circle A13 centre (-13.6739, 11.5) radius 0.7
  circle A14 centre (-11.1087, 11.5) radius 0.7
  circle A15 centre (-8.5435, 11.5) radius 0.7
  circle A16 centre (-5.9783, 11.5) radius 0.7
  circle A17 centre (-3.413, 11.5) radius 0.7
  circle A18 centre (-0.8478, 11.5) radius 0.7
  circle A19 centre (1.7174, 11.5) radius 0.7
  circle A20 centre (4.2826, 11.5) radius 0.7
  circle A21 centre (6.8478, 11.5) radius 0.7
  circle A22 centre (9.413, 11.5) radius 0.7
  circle A23 centre (11.9783, 11.5) radius 0.7
  circle A24 centre (14.5435, 11.5) radius 0.7
  circle A25 centre (17.1087, 11.5) radius 0.7
  circle A26 centre (19.6739, 11.5) radius 0.7
  circle A27 centre (22.2391, 11.5) radius 0.7
  circle A28 centre (24.8043, 11.5) radius 0.7
  circle A29 centre (27.3696, 11.5) radius 0.7
  circle A30 centre (29.9348, 11.5) radius 0.7
  circle A31 centre (32.5, 11.5) radius 0.7
  circle A32 centre (-26.5, 8.9444) radius 0.7
  circle A33 centre (-23.9348, 8.9444) radius 0.7
  circle A34 centre (-21.3696, 8.9444) radius 0.7
  circle A35 centre (-18.8043, 8.9444) radius 0.7
  circle A36 centre (-16.2391, 8.9444) radius 0.7
  circle A37 centre (-13.6739, 8.9444) radius 0.7
  circle A38 centre (-11.1087, 8.9444) radius 0.7
  circle A39 centre (-8.5435, 8.9444) radius 0.7
  circle A40 centre (-5.9783, 8.9444) radius 0.7
  circle A41 centre (-3.413, 8.9444) radius 0.7
  circle A42 centre (-0.8478, 8.9444) radius 0.7
  circle A43 centre (1.7174, 8.9444) radius 0.7
  circle A44 centre (4.2826, 8.9444) radius 0.7
  circle A45 centre (6.8478, 8.9444) radius 0.7
  circle A46 centre (9.413, 8.9444) radius 0.7
  circle A47 centre (11.9783, 8.9444) radius 0.7
  circle A48 centre (14.5435, 8.9444) radius 0.7
  circle A49 centre (17.1087, 8.9444) radius 0.7
  circle A50 centre (19.6739, 8.9444) radius 0.7
  circle A51 centre (22.2391, 8.9444) radius 0.7
  circle A52 centre (24.8043, 8.9444) radius 0.7
  circle A53 centre (27.3696, 8.9444) radius 0.7
  circle A54 centre (29.9348, 8.9444) radius 0.7
  circle A55 centre (32.5, 8.9444) radius 0.7
  circle A56 centre (-26.5, 6.3889) radius 0.7
  circle A57 centre (-23.9348, 6.3889) radius 0.7
  circle A58 centre (-21.3696, 6.3889) radius 0.7
  circle A59 centre (-18.8043, 6.3889) radius 0.7
  circle A60 centre (-16.2391, 6.3889) radius 0.7
  circle A61 centre (-13.6739, 6.3889) radius 0.7
  circle A62 centre (-11.1087, 6.3889) radius 0.7
  circle A63 centre (-8.5435, 6.3889) radius 0.7
  circle A64 centre (-5.9783, 6.3889) radius 0.7
  circle A65 centre (-3.413, 6.3889) radius 0.7
  circle A66 centre (-0.8478, 6.3889) radius 0.7
  circle A67 centre (1.7174, 6.3889) radius 0.7
  circle A68 centre (4.2826, 6.3889) radius 0.7
  circle A69 centre (6.8478, 6.3889) radius 0.7
  circle A70 centre (9.413, 6.3889) radius 0.7
  circle A71 centre (11.9783, 6.3889) radius 0.7
  circle A72 centre (14.5435, 6.3889) radius 0.7
  circle A73 centre (17.1087, 6.3889) radius 0.7
  circle A74 centre (19.6739, 6.3889) radius 0.7
  circle A75 centre (22.2391, 6.3889) radius 0.7
  circle A76 centre (24.8043, 6.3889) radius 0.7
  circle A77 centre (27.3696, 6.3889) radius 0.7
  circle A78 centre (29.9348, 6.3889) radius 0.7
  circle A79 centre (32.5, 6.3889) radius 0.7
  circle A80 centre (-26.5, 3.8333) radius 0.7
  circle A81 centre (-23.9348, 3.8333) radius 0.7
  circle A82 centre (-21.3696, 3.8333) radius 0.7
  circle A83 centre (-18.8043, 3.8333) radius 0.7
  circle A84 centre (-16.2391, 3.8333) radius 0.7
  circle A85 centre (-13.6739, 3.8333) radius 0.7
  circle A86 centre (-11.1087, 3.8333) radius 0.7
  circle A87 centre (-8.5435, 3.8333) radius 0.7
  circle A88 centre (-5.9783, 3.8333) radius 0.7
  circle A89 centre (-3.413, 3.8333) radius 0.7
  circle A90 centre (-0.8478, 3.8333) radius 0.7
  circle A91 centre (1.7174, 3.8333) radius 0.7
  circle A92 centre (4.2826, 3.8333) radius 0.7
  circle A93 centre (6.8478, 3.8333) radius 0.7
  circle A94 centre (9.413, 3.8333) radius 0.7
  circle A95 centre (11.9783, 3.8333) radius 0.7
  circle A96 centre (14.5435, 3.8333) radius 0.7
  circle A97 centre (17.1087, 3.8333) radius 0.7
  circle A98 centre (19.6739, 3.8333) radius 0.7
  circle A99 centre (22.2391, 3.8333) radius 0.7
  circle A100 centre (24.8043, 3.8333) radius 0.7
  circle A101 centre (27.3696, 3.8333) radius 0.7
  circle A102 centre (29.9348, 3.8333) radius 0.7
  circle A103 centre (32.5, 3.8333) radius 0.7
  circle A104 centre (-21.3696, 1.2778) radius 0.7
  circle A105 centre (-18.8043, 1.2778) radius 0.7
  circle A106 centre (-16.2391, 1.2778) radius 0.7
  circle A107 centre (-13.6739, 1.2778) radius 0.7
  circle A108 centre (-11.1087, 1.2778) radius 0.7
  circle A109 centre (-8.5435, 1.2778) radius 0.7
  circle A110 centre (-5.9783, 1.2778) radius 0.7
  circle A111 centre (-3.413, 1.2778) radius 0.7
  circle A112 centre (-0.8478, 1.2778) radius 0.7
  circle A113 centre (1.7174, 1.2778) radius 0.7
  circle A114 centre (4.2826, 1.2778) radius 0.7
  circle A115 centre (6.8478, 1.2778) radius 0.7
  circle A116 centre (9.413, 1.2778) radius 0.7
  circle A117 centre (11.9783, 1.2778) radius 0.7
  circle A118 centre (14.5435, 1.2778) radius 0.7
  circle A119 centre (17.1087, 1.2778) radius 0.7
  circle A120 centre (19.6739, 1.2778) radius 0.7
  circle A121 centre (22.2391, 1.2778) radius 0.7
  circle A122 centre (24.8043, 1.2778) radius 0.7
  circle A123 centre (27.3696, 1.2778) radius 0.7
  circle A124 centre (29.9348, 1.2778) radius 0.7
  circle A125 centre (32.5, 1.2778) radius 0.7
  circle A126 centre (-21.3696, -1.2778) radius 0.7
  circle A127 centre (-18.8043, -1.2778) radius 0.7
  circle A128 centre (-16.2391, -1.2778) radius 0.7
  circle A129 centre (-13.6739, -1.2778) radius 0.7
  circle A130 centre (-11.1087, -1.2778) radius 0.7
  circle A131 centre (-8.5435, -1.2778) radius 0.7
  circle A132 centre (-5.9783, -1.2778) radius 0.7
  circle A133 centre (-3.413, -1.2778) radius 0.7
  circle A134 centre (-0.8478, -1.2778) radius 0.7
  circle A135 centre (1.7174, -1.2778) radius 0.7
  circle A136 centre (4.2826, -1.2778) radius 0.7
  circle A137 centre (6.8478, -1.2778) radius 0.7
  circle A138 centre (9.413, -1.2778) radius 0.7
  circle A139 centre (11.9783, -1.2778) radius 0.7
  circle A140 centre (14.5435, -1.2778) radius 0.7
  circle A141 centre (17.1087, -1.2778) radius 0.7
  circle A142 centre (19.6739, -1.2778) radius 0.7
  circle A143 centre (22.2391, -1.2778) radius 0.7
  circle A144 centre (24.8043, -1.2778) radius 0.7
  circle A145 centre (27.3696, -1.2778) radius 0.7
  circle A146 centre (29.9348, -1.2778) radius 0.7
  circle A147 centre (32.5, -1.2778) radius 0.7
  circle A148 centre (-26.5, -3.8333) radius 0.7
  circle A149 centre (-23.9348, -3.8333) radius 0.7
  circle A150 centre (-21.3696, -3.8333) radius 0.7
  circle A151 centre (-18.8043, -3.8333) radius 0.7
  circle A152 centre (-16.2391, -3.8333) radius 0.7
  circle A153 centre (-13.6739, -3.8333) radius 0.7
  circle A154 centre (-11.1087, -3.8333) radius 0.7
  circle A155 centre (-8.5435, -3.8333) radius 0.7
  circle A156 centre (-5.9783, -3.8333) radius 0.7
  circle A157 centre (-3.413, -3.8333) radius 0.7
  circle A158 centre (-0.8478, -3.8333) radius 0.7
  circle A159 centre (1.7174, -3.8333) radius 0.7
  circle A160 centre (4.2826, -3.8333) radius 0.7
  circle A161 centre (6.8478, -3.8333) radius 0.7
  circle A162 centre (9.413, -3.8333) radius 0.7
  circle A163 centre (11.9783, -3.8333) radius 0.7
  circle A164 centre (14.5435, -3.8333) radius 0.7
  circle A165 centre (17.1087, -3.8333) radius 0.7
  circle A166 centre (19.6739, -3.8333) radius 0.7
  circle A167 centre (22.2391, -3.8333) radius 0.7
  circle A168 centre (24.8043, -3.8333) radius 0.7
  circle A169 centre (27.3696, -3.8333) radius 0.7
  circle A170 centre (29.9348, -3.8333) radius 0.7
  circle A171 centre (32.5, -3.8333) radius 0.7
  circle A172 centre (-26.5, -6.3889) radius 0.7
  circle A173 centre (-23.9348, -6.3889) radius 0.7
  circle A174 centre (-21.3696, -6.3889) radius 0.7
  circle A175 centre (-18.8043, -6.3889) radius 0.7
  circle A176 centre (-16.2391, -6.3889) radius 0.7
  circle A177 centre (-13.6739, -6.3889) radius 0.7
  circle A178 centre (-11.1087, -6.3889) radius 0.7
  circle A179 centre (-8.5435, -6.3889) radius 0.7
  circle A180 centre (-5.9783, -6.3889) radius 0.7
  circle A181 centre (-3.413, -6.3889) radius 0.7
  circle A182 centre (-0.8478, -6.3889) radius 0.7
  circle A183 centre (1.7174, -6.3889) radius 0.7
  circle A184 centre (4.2826, -6.3889) radius 0.7
  circle A185 centre (6.8478, -6.3889) radius 0.7
  circle A186 centre (9.413, -6.3889) radius 0.7
  circle A187 centre (11.9783, -6.3889) radius 0.7
  circle A188 centre (14.5435, -6.3889) radius 0.7
  circle A189 centre (17.1087, -6.3889) radius 0.7
  circle A190 centre (19.6739, -6.3889) radius 0.7
  circle A191 centre (22.2391, -6.3889) radius 0.7
  circle A192 centre (24.8043, -6.3889) radius 0.7
  circle A193 centre (27.3696, -6.3889) radius 0.7
  circle A194 centre (29.9348, -6.3889) radius 0.7
  circle A195 centre (32.5, -6.3889) radius 0.7
  circle A196 centre (-26.5, -8.9444) radius 0.7
  circle A197 centre (-23.9348, -8.9444) radius 0.7
  circle A198 centre (-21.3696, -8.9444) radius 0.7
  circle A199 centre (-18.8043, -8.9444) radius 0.7
  circle A200 centre (-16.2391, -8.9444) radius 0.7
  circle A201 centre (-13.6739, -8.9444) radius 0.7
  circle A202 centre (-11.1087, -8.9444) radius 0.7
  circle A203 centre (-8.5435, -8.9444) radius 0.7
  circle A204 centre (-5.9783, -8.9444) radius 0.7
  circle A205 centre (-3.413, -8.9444) radius 0.7
  circle A206 centre (-0.8478, -8.9444) radius 0.7
  circle A207 centre (1.7174, -8.9444) radius 0.7
  circle A208 centre (4.2826, -8.9444) radius 0.7
  circle A209 centre (6.8478, -8.9444) radius 0.7
  circle A210 centre (9.413, -8.9444) radius 0.7
  circle A211 centre (11.9783, -8.9444) radius 0.7
  circle A212 centre (14.5435, -8.9444) radius 0.7
  circle A213 centre (17.1087, -8.9444) radius 0.7
  circle A214 centre (19.6739, -8.9444) radius 0.7
  circle A215 centre (22.2391, -8.9444) radius 0.7
  circle A216 centre (24.8043, -8.9444) radius 0.7
  circle A217 centre (27.3696, -8.9444) radius 0.7
  circle A218 centre (29.9348, -8.9444) radius 0.7
  circle A219 centre (32.5, -8.9444) radius 0.7
  circle A220 centre (-26.5, -11.5) radius 0.7
  circle A221 centre (-23.9348, -11.5) radius 0.7
  circle A222 centre (-21.3696, -11.5) radius 0.7
  circle A223 centre (-18.8043, -11.5) radius 0.7
  circle A224 centre (-16.2391, -11.5) radius 0.7
  circle A225 centre (-13.6739, -11.5) radius 0.7
  circle A226 centre (-11.1087, -11.5) radius 0.7
  circle A227 centre (-8.5435, -11.5) radius 0.7
  circle A228 centre (-5.9783, -11.5) radius 0.7
  circle A229 centre (-3.413, -11.5) radius 0.7
  circle A230 centre (-0.8478, -11.5) radius 0.7
  circle A231 centre (1.7174, -11.5) radius 0.7
  circle A232 centre (4.2826, -11.5) radius 0.7
  circle A233 centre (6.8478, -11.5) radius 0.7
  circle A234 centre (9.413, -11.5) radius 0.7
  circle A235 centre (11.9783, -11.5) radius 0.7
  circle A236 centre (14.5435, -11.5) radius 0.7
  circle A237 centre (17.1087, -11.5) radius 0.7
  circle A238 centre (19.6739, -11.5) radius 0.7
  circle A239 centre (22.2391, -11.5) radius 0.7
  circle A240 centre (24.8043, -11.5) radius 0.7
  circle A241 centre (27.3696, -11.5) radius 0.7
  circle A242 centre (29.9348, -11.5) radius 0.7
  circle A243 centre (32.5, -11.5) radius 0.7
  circle A244 centre (-30, 13.1) radius 1.2
  circle A245 centre (36, 13.1) radius 1.2
  circle A246 centre (-30, -13.1) radius 1.2
  circle A247 centre (36, -13.1) radius 1.2
  line L8 (38, 15) -> (-32, 15)
  line L9 (38, -15) -> (38, 15)
  line L10 (-32, -15) -> (38, -15)
  line L11 (-32, 15) -> (-32, -15)
  line L12 (-26.5, -11.5) -> (-26.5, 0) construction
  line L13 (-26.5, 11.5) -> (-26.5, 0) construction
  circle A248 centre (-26.5, 0) radius 2.55
  point P0 (-26.5, 0)
  dimension "d225" = 5.1
  constraint coincident A220.centre L12.start
  constraint coincident P0 L12.end
  constraint vertical L12
  constraint coincident A8.centre L13.start
  constraint equal L12 L13
  measures "d225" diameter of A248